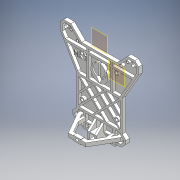
# Autodesk Inventor part: Base_v6
Saved by Autodesk Inventor 2016 (Build 200138000, 138)
## iProperties
Created: 2015-10-26
Part Number: Base_v6
Material: Generic
Document SubType Name: Modeling
Designer: Jared
Density: 1 g/cm^3
Appearance: Default
Author: Jared
Autodesk Inventor part; units mm, degrees
(part 1 of 2)
ref_plane "YZ Plane" through (0, 0, 0) normal (1, 0, 0) x (0, 1, 0)
ref_plane "XZ Plane" through (0, 0, 0) normal (0, 1, 0) x (-1, 0, 0)
ref_plane "XY Plane" through (0, 0, 0) normal (0, 0, 1) x (1, 0, 0)
sketch "Block1" plane through (0, 0, 0) normal (0, 0, 1) x (1, 0, 0)
  line L0 (52, 0) -> (42, 0)
  line L1 (52, 0) -> (56.9992, -4.9992)
  line L2 (52, 0) -> (59.07, 0) construction
  line L3 (56.9992, -4.9992) -> (56.9992, -14.9992)
  point P0 (53.472, -3.4612)
sketch "OuterRim" plane through (0, 0, 0) normal (0, 0, 1) x (1, 0, 0)
  line L0 (39.5, 1) -> (24.5001, -13.9999)
  line L1 (24.5001, -13.9999) -> (0.0001, -13.9999)
  line L2 (54.5031, -13.9999) -> (32.0031, -52.971)
  line L3 (32.0031, -52.971) -> (32.0031, -111.471)
  line L4 (32.0031, -111.471) -> (37.0024, -116.4702)
  line L5 (37.0024, -121.4734) -> (32.0002, -126.4756)
  line L6 (37.0024, -121.4734) -> (37.0024, -116.4702)
  line L7 (22.0011, -131.4748) -> (0.0003, -131.4748)
  line L8 (32.0002, -126.4756) -> (30.5003, -127.9756)
  line L9 (30.5003, -127.9756) -> (25.5003, -127.9756)
  line L10 (25.5003, -127.9756) -> (22.0011, -131.4748)
  line L11 (-36.9986, -121.4763) -> (-31.9993, -126.4756)
  line L12 (-36.9986, -121.4763) -> (-36.9986, -116.4706)
  line L13 (-31.9993, -126.4756) -> (-30.4993, -127.9756)
  line L14 (-22.0002, -131.4748) -> (0.0003, -131.4748)
  line L15 (-31.999, -111.471) -> (-36.9986, -116.4706)
  line L16 (-30.4993, -127.9756) -> (-25.4993, -127.9756)
  line L17 (-25.4993, -127.9756) -> (-22.0002, -131.4748)
  line L18 (-31.999, -52.971) -> (-31.999, -111.471)
  line L19 (-39.4997, 1) -> (-24.4999, -13.9999)
  line L20 (-24.4999, -13.9999) -> (0.0001, -13.9999)
  line L21 (-54.499, -13.9999) -> (-31.999, -52.971)
  line L22 (49.5, 1) -> (39.5, 1)
  line L23 (49.5, 1) -> (54.4992, -3.9992)
  line L24 (49.5, 1) -> (56.57, 1) construction
  line L25 (54.4992, -3.9992) -> (54.4992, -13.9992)
  line L26 (-49.4997, 1) -> (-39.4997, 1)
  line L27 (-49.4997, 1) -> (-54.499, -3.9992)
  line L28 (-49.4997, 1) -> (-56.5697, 1) construction
  line L29 (-54.499, -3.9992) -> (-54.499, -13.9992)
  point P0 (0.0001, -89.0989)
sketch "OuterRim1" plane through (0, 0, 0) normal (0, 0, 1) x (1, 0, 0)
  line L0 (-39.4997, 1) -> (-24.4999, -13.9998)
  line L1 (-24.4999, -13.9998) -> (0.0001, -13.9998)
  line L2 (-54.499, -13.9998) -> (-31.999, -52.971)
  line L3 (-31.999, -52.971) -> (-31.999, -111.471)
  line L4 (-31.999, -111.471) -> (-36.9986, -116.4706)
  line L5 (-36.9986, -121.4763) -> (-31.9993, -126.4756)
  line L6 (-36.9986, -121.4763) -> (-36.9986, -116.4706)
  line L7 (-22.0002, -131.4747) -> (0.0003, -131.4747)
  line L8 (-31.9993, -126.4756) -> (-30.4993, -127.9756)
  line L9 (-30.4993, -127.9756) -> (-25.4993, -127.9756)
  line L10 (-25.4993, -127.9756) -> (-22.0002, -131.4747)
  line L11 (39.5, 1) -> (24.5001, -13.9998)
  line L12 (24.5001, -13.9998) -> (0.0001, -13.9998)
  line L13 (32.0002, -126.4756) -> (30.5003, -127.9756)
  line L14 (30.5003, -127.9756) -> (25.5003, -127.9756)
  line L15 (25.5003, -127.9756) -> (22.0011, -131.4747)
  line L16 (54.5031, -13.9998) -> (32.0031, -52.971)
  line L17 (32.0031, -52.971) -> (32.0031, -111.471)
  line L18 (32.0031, -111.471) -> (37.0024, -116.4702)
  line L19 (37.0024, -121.4734) -> (32.0002, -126.4756)
  line L20 (37.0024, -121.4734) -> (37.0024, -116.4702)
  line L21 (22.0011, -131.4747) -> (0.0003, -131.4747)
  line L22 (49.5, 1) -> (39.5, 1)
  line L23 (49.5, 1) -> (54.5031, -3.9992)
  line L24 (54.5031, -3.9992) -> (54.5031, -13.9998)
  line L25 (-49.4997, 1) -> (-39.4997, 1)
  line L26 (-49.4997, 1) -> (-54.499, -3.9992)
  line L27 (-54.499, -3.9992) -> (-54.499, -13.9998)
  point P0 (0.0008, -71.4203)
sketch "outerrim2" plane through (0, 0, 0) normal (0, 0, 1) x (1, 0, 0)
  line L0 (49.5, 1) -> (39.5, 1)
  line L1 (49.5, 1) -> (54.5012, -3.9973)
  line L2 (54.5012, -3.9973) -> (54.5012, -13.9979)
  line L3 (-49.4997, 1) -> (-39.4997, 1)
  line L4 (-49.4997, 1) -> (-54.499, -3.9992)
  line L5 (-54.499, -3.9992) -> (-54.499, -13.9998)
  line L6 (-39.4997, 1) -> (-24.4999, -13.9998)
  line L7 (-24.4999, -13.9998) -> (0.0001, -13.9998)
  line L8 (-54.499, -13.9998) -> (-31.999, -52.971)
  line L9 (-31.999, -101.471) -> (-36.9986, -106.4706)
  line L10 (-36.9986, -111.4763) -> (-31.9993, -116.4756)
  line L11 (-36.9986, -111.4763) -> (-36.9986, -106.4706)
  line L12 (-22.0002, -121.4747) -> (0.0003, -121.4747)
  line L13 (-31.9993, -116.4756) -> (-30.4993, -117.9756)
  line L14 (-30.4993, -117.9756) -> (-25.4993, -117.9756)
  line L15 (-25.4993, -117.9756) -> (-22.0002, -121.4747)
  line L16 (39.5, 1) -> (24.5001, -13.9998)
  line L17 (24.5001, -13.9998) -> (0.0001, -13.9998)
  line L18 (32.0002, -116.4756) -> (30.5003, -117.9756)
  line L19 (30.5003, -117.9756) -> (25.5003, -117.9756)
  line L20 (25.5003, -117.9756) -> (22.0011, -121.4747)
  line L21 (54.5012, -13.9979) -> (32.0031, -52.971)
  line L22 (32.0031, -101.471) -> (37.0024, -106.4702)
  line L23 (37.0024, -111.4734) -> (32.0002, -116.4756)
  line L24 (37.0024, -111.4734) -> (37.0024, -106.4702)
  line L25 (22.0011, -121.4747) -> (0.0003, -121.4747)
  line L26 (-31.999, -52.971) -> (-31.999, -101.471)
  line L27 (32.0031, -52.971) -> (32.0031, -101.471)
  point P0 (0.0009, -67.4302)
sketch "Sketch1" plane through (0, 0, 0) normal (0, 1, 0) x (-1, 0, 0)
  line L0 (24.9992, -101.4702) -> (24.9992, -106.4702)
  line L1 (24.9992, -101.4702) -> (29.9992, -101.4702)
  line L2 (29.9992, -101.4702) -> (29.9992, -106.4702)
  line L3 (29.9992, -106.4702) -> (24.9992, -106.4702)
  line L4 (22.0008, -108.476) -> (24.9999, -111.4752)
  line L5 (22.0008, -114.4744) -> (24.9999, -111.4752)
  line L6 (33.9992, -105.2276) -> (30.7516, -108.4752)
  line L7 (33.9992, -103.2094) -> (33.9992, -105.2276)
  line L8 (29.9986, -51.0238) -> (29.1311, -53.1497)
  line L9 (51.4221, -5.197) -> (51.4221, -13.955)
  line L10 (48.1802, -1.9551) -> (51.4221, -5.197)
  line L11 (26.5443, -16.0763) -> (40.6655, -1.9551)
  line L12 (40.6655, -1.9551) -> (48.1802, -1.9551)
  line L13 (24.423, -16.955) -> (26.5443, -16.0763)
  line L14 (0.0001, -13.9999) -> (3.0001, -13.9999) construction
  line L15 (15.5025, -107.9762) -> (12.7427, -110.1594)
  line L16 (6.5073, -114.9942) -> (11.0731, -111.4803)
  line L17 (13.1989, -114.9663) -> (15.569, -114.9604)
  line L18 (13.1989, -114.9663) -> (9.927, -114.9744)
  line L19 (9.927, -114.9744) -> (12.7467, -112.7943)
  line L20 (9.927, -114.9744) -> (13.4912, -114.9744) construction
  line L21 (18.978, -107.9762) -> (14.4463, -111.4804)
  line L22 (14.4463, -111.4804) -> (18.978, -114.9745)
  line L23 (12.7427, -110.1594) -> (9.9014, -107.9762)
  line L24 (11.0731, -111.4803) -> (6.5073, -107.976)
  line L25 (12.7467, -112.7943) -> (15.569, -114.9604)
  line L26 (22.0008, -106.476) -> (23.9999, -108.4752)
  line L27 (22.0008, -108.476) -> (22.0008, -114.4744)
  line L28 (18.978, -107.9762) -> (18.978, -114.9745)
  line L29 (6.5073, -107.976) -> (6.5073, -114.9942)
  line L30 (3.5, -108.0056) -> (3.5, -115.0056)
  circle A0 centre (39.4726, -5.9876) radius 1.1
  circle A1 centre (30.4217, -15.0386) radius 1.1
  line L31 (30.7516, -108.4752) -> (29.2517, -109.9752)
  line L32 (23.9999, -108.4752) -> (25.4999, -109.9752)
  line L33 (25.4999, -109.9752) -> (29.2517, -109.9752)
  line L34 (33.9992, -103.2094) -> (29, -98.2258)
  line L35 (29, -98.2258) -> (29, -96.471)
  circle A2 centre (23.9999, -27) radius 1.5
  circle A3 centre (23.9999, -83) radius 1.5
  line L36 (9.5, -55.971) -> (18.4788, -64.9632)
  line L37 (20.0067, -66.4933) -> (29, -75.5)
  line L38 (7.9989, -57.4721) -> (16.9989, -66.4855)
  line L39 (18.5056, -67.9944) -> (27.4978, -77)
  line L40 (27.471, -55.971) -> (18.4788, -64.9632)
  line L41 (20.0067, -66.4933) -> (29, -57.5)
  line L42 (29, -57.5) -> (29, -75.5)
  line L43 (27.471, -55.971) -> (9.5, -55.971)
  line L44 (6.5, -55.971) -> (0.0001, -55.971)
  line L45 (29.1311, -53.1497) -> (18.1317, -53.2075)
  line L46 (15, -52.971) -> (0.0001, -52.971)
  line L47 (24.423, -16.955) -> (18, -16.955)
  line L48 (15, -16.9999) -> (0.0001, -16.9999)
  line L49 (22.0008, -106.476) -> (22.0008, -96.471)
  line L50 (19.0008, -106.476) -> (19.0008, -96.471)
  line L51 (3.5, -106.476) -> (3.5, -96.471)
  line L52 (6.5, -106.476) -> (6.5, -96.471)
  line L53 (6.5, -106.476) -> (19.0008, -106.476)
  line L54 (22.0008, -96.471) -> (29, -96.471)
  line L55 (19.0008, -96.471) -> (6.5, -96.471)
  line L56 (18, -28.1451) -> (18.1317, -53.2075)
  line L57 (15, -28) -> (15, -52.971)
  line L58 (43.2847, -28.1039) -> (29.9986, -51.0238)
  line L59 (-24.999, -101.4702) -> (-24.999, -106.4702)
  line L60 (-24.999, -101.4702) -> (-29.999, -101.4702)
  line L61 (-29.999, -101.4702) -> (-29.999, -106.4702)
  line L62 (-29.999, -106.4702) -> (-24.999, -106.4702)
  line L63 (-22.0005, -108.476) -> (-24.9996, -111.4752)
  line L64 (-22.0005, -114.4744) -> (-24.9996, -111.4752)
  line L65 (-33.999, -105.2276) -> (-30.7514, -108.4752)
  line L66 (-33.999, -103.2094) -> (-33.999, -105.2276)
  line L67 (-29.8784, -50.8497) -> (-28.9997, -52.971)
  line L68 (-51.4218, -5.197) -> (-51.4218, -13.955)
  line L69 (-48.1799, -1.9551) -> (-51.4218, -5.197)
  line L70 (-26.544, -16.0763) -> (-40.6652, -1.9551)
  line L71 (-40.6652, -1.9551) -> (-48.1799, -1.9551)
  line L72 (-24.4227, -16.955) -> (-26.544, -16.0763)
  line L73 (0.0001, -13.9999) -> (-2.9999, -13.9999) construction
  line L74 (-15.5021, -107.976) -> (-12.7423, -110.1593)
  line L75 (-6.5069, -114.9941) -> (-11.0727, -111.4802)
  line L76 (-13.1987, -114.9663) -> (-15.5687, -114.9604)
  line L77 (-13.1987, -114.9663) -> (-9.9267, -114.9744)
  line L78 (-9.9267, -114.9744) -> (-12.7464, -112.7943)
  line L79 (-9.9267, -114.9744) -> (-13.4909, -114.9744) construction
  line L80 (-18.9776, -107.976) -> (-14.4459, -111.4803)
  line L81 (-14.4459, -111.4803) -> (-18.9776, -114.9744)
  line L82 (-12.7423, -110.1593) -> (-9.901, -107.976)
  line L83 (-11.0727, -111.4802) -> (-6.5069, -107.9759)
  line L84 (-12.7464, -112.7943) -> (-15.5687, -114.9604)
  line L85 (-22.0005, -106.476) -> (-23.9996, -108.4752)
  line L86 (-22.0005, -108.476) -> (-22.0005, -114.4744)
  line L87 (-18.9776, -107.976) -> (-18.9776, -114.9744)
  line L88 (-6.5069, -107.9759) -> (-6.5069, -114.9941)
  line L89 (-3.4997, -108.0056) -> (-3.4997, -115.0056)
  circle A4 centre (-39.4723, -5.9876) radius 1.1
  circle A5 centre (-30.4214, -15.0386) radius 1.1
  line L90 (-30.7514, -108.4752) -> (-29.2514, -109.9752)
  line L91 (-23.9996, -108.4752) -> (-25.4997, -109.9752)
  line L92 (-25.4997, -109.9752) -> (-29.2514, -109.9752)
  line L93 (-33.999, -103.2094) -> (-28.9997, -98.2258)
  line L94 (-28.9997, -98.2258) -> (-28.9997, -96.471)
  circle A6 centre (-23.9996, -27) radius 1.5
  circle A7 centre (-23.9996, -83) radius 1.5
  line L95 (-9.4997, -55.971) -> (-18.4785, -64.9632)
  line L96 (-20.0064, -66.4933) -> (-28.9997, -75.5)
  line L97 (-7.9986, -57.4721) -> (-16.9986, -66.4855)
  line L98 (-18.5053, -67.9945) -> (-27.4975, -77.0001)
  line L99 (-27.4707, -55.971) -> (-18.4785, -64.9632)
  line L100 (-20.0064, -66.4933) -> (-28.9997, -57.5)
  line L101 (-28.9997, -57.5) -> (-28.9997, -75.5)
  line L102 (-27.4707, -55.971) -> (-9.4997, -55.971)
  line L103 (-6.4997, -55.971) -> (0.0001, -55.971)
  line L104 (-28.9997, -52.971) -> (-17.9997, -52.971)
  line L105 (-14.9997, -52.971) -> (0.0001, -52.971)
  line L106 (-24.4227, -16.955) -> (-17.9997, -16.955)
  line L107 (-14.9997, -16.9999) -> (0.0001, -16.9999)
  line L108 (-22.0005, -106.476) -> (-22.0005, -96.471)
  line L109 (-19.0005, -106.476) -> (-19.0005, -96.471)
  line L110 (-3.4997, -106.476) -> (-3.4997, -96.471)
  line L111 (-6.4997, -106.476) -> (-6.4997, -96.471)
  line L112 (-6.4997, -106.476) -> (-19.0005, -106.476)
  line L113 (-22.0005, -96.471) -> (-28.9997, -96.471)
  line L114 (-19.0005, -96.471) -> (-6.4997, -96.471)
  line L115 (-17.9997, -28) -> (-17.9997, -52.971)
  line L116 (-14.9997, -28) -> (-14.9997, -52.971)
  line L117 (-51.4218, -13.955) -> (-45.0449, -25)
  line L118 (-43.2848, -28) -> (-29.8784, -50.8497)
  line L119 (54.5012, -13.9979) -> (54.4973, -13.9973)
  line L120 (3.5, -115.0056) -> (-3.4997, -115.0056)
  line L121 (3.5, -96.471) -> (-3.4997, -96.471)
  line L122 (49.5, 1) -> (56.57, 1) construction
  line L123 (-49.4997, 1) -> (-56.5697, 1) construction
  line L124 (-15.5021, -107.976) -> (-9.901, -107.976)
  line L125 (15.5025, -107.9762) -> (9.9014, -107.9762)
  line L126 (-17.9997, -21) -> (-47.3543, -21)
  line L127 (-17.9997, -16.955) -> (-17.9997, -21)
  line L128 (-14.9997, -16.9999) -> (-14.9997, -21)
  line L129 (15, -21) -> (-14.9997, -21)
  line L130 (15, -16.9999) -> (15, -21)
  line L131 (18, -21) -> (18, -16.955)
  line L132 (18, -21) -> (47.3546, -21)
  line L133 (51.4221, -13.955) -> (47.3546, -21)
  line L134 (45.6012, -24.0917) -> (43.2847, -28.1039)
  line L135 (18, -28.1451) -> (18, -24.0917)
  line L136 (-17.9997, -24) -> (-45.6223, -24)
  line L137 (15, -24) -> (15, -28)
  line L138 (-14.9997, -24) -> (-14.9997, -28)
  line L139 (-17.9997, -28) -> (-17.9997, -24)
  circle A8 centre (-46.9997, -6.5) radius 2
  circle A9 centre (47, -6.5) radius 2
  circle A10 centre (-23.9996, -27) radius 3
  arc A11 (-21.0442, -83.5154) -> (-23.4842, -85.9554) centre (-23.9996, -83) ccw
  arc A12 (23.2638, -24.0917) -> (24.7361, -24.0917) centre (23.9999, -27) ccw
  arc A13 (23.4849, -85.9555) -> (21.0445, -83.515) centre (23.9999, -83) ccw
  circle A14 centre (30.4217, -15.0386) radius 2
  circle A15 centre (39.4726, -5.9876) radius 2
  circle A16 centre (-30.4214, -15.0386) radius 2
  circle A17 centre (-39.4723, -5.9876) radius 2
  line L140 (1, -29) -> (1, -42.9373)
  line L141 (-1, -29) -> (-1, -42.9372)
  line L142 (0, -50.9997) -> (-3.9281, -44.1961)
  line L143 (0, -50.9997) -> (3.9287, -44.1961)
  line L144 (-45.0449, -25) -> (-43.2848, -28)
  line L145 (-14.9997, -24) -> (15, -24)
  line L146 (-3.4997, -106.476) -> (3.5, -106.476)
  line L147 (-3.4997, -108.0056) -> (3.5, -108.0056)
  arc A18 (-9.367, -31.4996) -> (9.3679, -31.5004) centre (0.0001, -39) ccw
  arc A19 (-9.367, -31.4996) -> (-3.9281, -44.1961) centre (0.0003, -35) ccw
  arc A20 (3.9287, -44.1961) -> (9.3679, -31.5004) centre (0.0003, -35) ccw
  line L148 (-1, -29) -> (-1, -27.0628)
  line L149 (1, -29) -> (1, -27.0627)
  arc A21 (1, -42.9373) -> (1, -27.0627) centre (0.0003, -35) ccw
  arc A22 (-1, -27.0628) -> (-1, -42.9372) centre (0.0003, -35) ccw
  line L150 (49.5, 1) -> (39.5, 1)
  line L151 (49.5, 1) -> (54.5012, -3.9973)
  line L152 (54.5012, -3.9973) -> (54.5012, -13.9979)
  line L153 (-49.4997, 1) -> (-39.4997, 1)
  line L154 (-39.4997, 1) -> (-24.4999, -13.9998)
  line L155 (-24.4999, -13.9998) -> (0.0001, -13.9998)
  line L156 (-31.999, -96.471) -> (-36.9986, -101.4706)
  line L157 (-36.9986, -106.4763) -> (-31.9993, -111.4756)
  line L158 (-36.9986, -106.4763) -> (-36.9986, -101.4706)
  line L159 (-22.0002, -116.4747) -> (0.0003, -116.4747)
  line L160 (-31.9993, -111.4756) -> (-30.4993, -112.9756)
  line L161 (-30.4993, -112.9756) -> (-25.4993, -112.9756)
  line L162 (-25.4993, -112.9756) -> (-22.0002, -116.4747)
  line L163 (39.5, 1) -> (24.5001, -13.9998)
  line L164 (24.5001, -13.9998) -> (0.0001, -13.9998)
  line L165 (32.0002, -111.4756) -> (30.5003, -112.9756)
  line L166 (30.5003, -112.9756) -> (25.5003, -112.9756)
  line L167 (25.5003, -112.9756) -> (22.0011, -116.4747)
  line L168 (54.5012, -13.9979) -> (32.0031, -52.971)
  line L169 (32.0031, -96.471) -> (37.0024, -101.4702)
  line L170 (37.0024, -106.4734) -> (32.0002, -111.4756)
  line L171 (37.0024, -106.4734) -> (37.0024, -101.4702)
  line L172 (22.0011, -116.4747) -> (0.0003, -116.4747)
  line L173 (-49.4997, 1) -> (-54.499, -3.9992)
  line L174 (-54.499, -3.9992) -> (-54.499, -13.9998)
  line L175 (-54.499, -13.9998) -> (-31.999, -52.971)
  line L176 (-31.999, -52.971) -> (-31.999, -96.471)
  line L177 (32.0031, -52.971) -> (32.0031, -96.471)
  line L178 (29, -78.5022) -> (29, -91.4705)
  line L179 (-28.9997, -78.5045) -> (-28.9997, -91.4709)
  line L180 (-27.4975, -77.0001) -> (-28.9997, -78.5045)
  line L181 (-28.0288, -93.5) -> (28.0295, -93.5)
  line L182 (27.4978, -77) -> (29, -78.5022)
  line L183 (23.4849, -85.9555) -> (29, -91.4705)
  line L184 (-23.4842, -85.9554) -> (-28.9997, -91.4709)
  line L185 (-10.5143, -75.9855) -> (-28.0288, -93.5)
  line L186 (-16.9986, -66.4855) -> (-10.4934, -72.9645)
  line L187 (-8.9904, -74.4615) -> (-6.4417, -77)
  line L188 (-12.0144, -74.4855) -> (-21.0442, -83.5154)
  line L189 (-9.4997, -77.0001) -> (-10.5143, -75.9855)
  line L190 (-12.0144, -74.4855) -> (-18.5053, -67.9945)
  line L191 (-7.9986, -57.4721) -> (-1.4998, -63.9709)
  line L192 (6.5, -55.971) -> (0.0002, -62.4709)
  line L193 (-1.4998, -63.9709) -> (-10.4934, -72.9645)
  line L194 (-6.4997, -55.971) -> (0.0002, -62.4709)
  line L195 (7.9989, -57.4721) -> (1.5002, -63.9709)
  line L196 (0.0002, -65.4709) -> (-8.9904, -74.4615)
  line L197 (16.9989, -66.4855) -> (10.4938, -72.9644)
  line L198 (8.9908, -74.4614) -> (6.442, -77)
  line L199 (9.5, -77) -> (10.5147, -75.9853)
  line L200 (12.0147, -74.4853) -> (18.5056, -67.9944)
  line L201 (0.0002, -65.4709) -> (8.9908, -74.4614)
  line L202 (10.5147, -75.9853) -> (28.0295, -93.5)
  line L203 (1.5002, -63.9709) -> (10.4938, -72.9644)
  line L204 (12.0147, -74.4853) -> (21.0445, -83.515)
  line L205 (-6.4417, -77) -> (0.0002, -83.4419)
  line L206 (1.5292, -84.9709) -> (10.0584, -93.5)
  line L207 (-9.4997, -77.0001) -> (-1.5289, -84.9709)
  line L208 (0.0002, -86.4999) -> (7.0003, -93.5)
  line L209 (6.442, -77) -> (0.0002, -83.4419)
  line L210 (-1.5289, -84.9709) -> (-10.0579, -93.5)
  line L211 (9.5, -77) -> (1.5292, -84.9709)
  line L212 (0.0002, -86.4999) -> (-6.9999, -93.5)
  line L213 (18, -24.0917) -> (23.2638, -24.0917)
  line L214 (24.7361, -24.0917) -> (45.6012, -24.0917)
  constraints: 433 end point, 30 parallel, 23 centre point, 16 point on circle, 15 horizontal, 14 point on line, 13 perpendicular, 9 coincident, 8 vertical, 1 collinear, 1 equal length
ref_plane "Work Plane3" through (0, 0, 0) normal (0, -1, 0) x (1, 0, 0)
sketch "Sketch8" plane through (0, 0, 0) normal (0, -1, 0) x (1, 0, 0)
  line L0 (49.5, 1) -> (39.5, 1)
  line L1 (49.5, 1) -> (54.5012, -3.9973)
  line L2 (54.5012, -3.9973) -> (54.5012, -13.9979)
  line L3 (-49.4997, 1) -> (-39.4997, 1)
  line L4 (-49.4997, 1) -> (-54.499, -3.9992)
  line L5 (-54.499, -3.9992) -> (-54.499, -13.9999)
  line L6 (-39.4997, 1) -> (-24.4999, -13.9999)
  line L7 (-24.4999, -13.9999) -> (0.0001, -13.9999)
  line L8 (-54.499, -13.9999) -> (-31.999, -52.971)
  line L9 (-31.999, -96.471) -> (-36.9986, -101.4706)
  line L10 (-36.9986, -106.4763) -> (-31.9993, -111.4756)
  line L11 (-36.9986, -106.4763) -> (-36.9986, -101.4706)
  line L12 (-22.0002, -116.4748) -> (0.0003, -116.4748)
  line L13 (-31.9993, -111.4756) -> (-30.4993, -112.9756)
  line L14 (-30.4993, -112.9756) -> (-25.4993, -112.9756)
  line L15 (-25.4993, -112.9756) -> (-22.0002, -116.4748)
  line L16 (39.5, 1) -> (24.5001, -13.9999)
  line L17 (24.5001, -13.9999) -> (0.0001, -13.9999)
  line L18 (32.0002, -111.4756) -> (30.5003, -112.9756)
  line L19 (30.5003, -112.9756) -> (25.5003, -112.9756)
  line L20 (25.5003, -112.9756) -> (22.0011, -116.4748)
  line L21 (54.5012, -13.9979) -> (32.0031, -52.971)
  line L22 (32.0031, -96.471) -> (37.0024, -101.4702)
  line L23 (37.0024, -106.4734) -> (32.0002, -111.4756)
  line L24 (37.0024, -106.4734) -> (37.0024, -101.4702)
  line L25 (22.0011, -116.4748) -> (0.0003, -116.4748)
  line L26 (32.0031, -52.971) -> (32.0031, -96.471)
  line L27 (-31.999, -96.471) -> (-31.999, -52.971)
  point P0 (0, 0)
  constraints: 56 end point, 4 horizontal, 2 vertical, 1 parallel, 1 perpendicular
ref_plane "Work Plane8" through (23.9996, 0, -27) normal (0, -1, 0) x (1, 0, 0)
sketch "Sketch10" plane through (23.9996, 0, -27) normal (0, -1, 0) x (1, 0, 0)
  circle A0 centre (0.0003, 0) radius 1.5 projected
  circle A1 centre (0.0003, 0) radius 1.5
  circle A2 centre (-47.9993, 0) radius 1.5 projected
  circle A3 centre (-47.9993, 0) radius 1.5
  circle A4 centre (-47.9993, 0) radius 2.9998
  circle A5 centre (-47.9996, -56) radius 3 projected
  circle A6 centre (-47.9996, -56) radius 1.5001
  circle A7 centre (-47.9996, -56) radius 3
  arc A8 (-0.0236, -53.0001) -> (0.0236, -53.0001) centre (0, -56) ccw projected
  circle A9 centre (0, -56) radius 1.5
  circle A10 centre (0, -56) radius 3
  circle A11 centre (0.0003, 0) radius 3
  circle A12 centre (0.0003, 0) radius 1.5
  point P0 (-23.9996, 27)
  dimension "d136" = 3
  constraints: 9 centre point, 9 coincident
  measures "d136" diameter of A1
sketch "Sketch20" plane through (0, 0, 0) normal (0, -1, 0) x (1, 0, 0)
  line L0 (24.9992, -101.4702) -> (24.9992, -106.4702)
  line L1 (24.9992, -101.4702) -> (29.9992, -101.4702)
  line L2 (29.9992, -101.4702) -> (29.9992, -106.4702)
  line L3 (29.9992, -106.4702) -> (24.9992, -106.4702)
  line L4 (22.0008, -108.476) -> (24.9999, -111.4752)
  line L5 (22.0008, -114.4744) -> (24.9999, -111.4752)
  line L6 (33.9992, -105.2276) -> (30.7516, -108.4752)
  line L7 (33.9992, -103.2094) -> (33.9992, -105.2276)
  line L8 (29.9986, -51.0238) -> (29.1311, -53.1497)
  line L9 (51.4221, -5.197) -> (51.4221, -13.955)
  line L10 (48.1802, -1.9551) -> (51.4221, -5.197)
  line L11 (26.5443, -16.0763) -> (40.6655, -1.9551)
  line L12 (40.6655, -1.9551) -> (48.1802, -1.9551)
  line L13 (24.423, -16.955) -> (26.5443, -16.0763)
  line L14 (0.0001, -13.9999) -> (3.0001, -13.9999) construction
  line L15 (15.5025, -107.9762) -> (12.7427, -110.1594)
  line L16 (6.5073, -114.9942) -> (11.0731, -111.4803)
  line L17 (13.1989, -114.9663) -> (15.569, -114.9604)
  line L18 (13.1989, -114.9663) -> (9.927, -114.9744)
  line L19 (9.927, -114.9744) -> (12.7467, -112.7943)
  line L20 (9.927, -114.9744) -> (13.4912, -114.9744) construction
  line L21 (18.978, -107.9762) -> (14.4463, -111.4804)
  line L22 (14.4463, -111.4804) -> (18.978, -114.9745)
  line L23 (12.7427, -110.1594) -> (9.9014, -107.9762)
  line L24 (11.0731, -111.4803) -> (6.5073, -107.976)
  line L25 (12.7467, -112.7943) -> (15.569, -114.9604)
  line L26 (22.0008, -106.476) -> (23.9999, -108.4752)
  line L27 (22.0008, -108.476) -> (22.0008, -114.4744)
  line L28 (18.978, -107.9762) -> (18.978, -114.9745)
  line L29 (6.5073, -107.976) -> (6.5073, -114.9942)
  line L30 (3.5, -108.0056) -> (3.5, -115.0056)
  circle A0 centre (39.4726, -5.9876) radius 1.1
  circle A1 centre (30.4217, -15.0386) radius 1.1
  line L31 (30.7516, -108.4752) -> (29.2517, -109.9752)
  line L32 (23.9999, -108.4752) -> (25.4999, -109.9752)
  line L33 (25.4999, -109.9752) -> (29.2517, -109.9752)
  line L34 (33.9992, -103.2094) -> (29, -98.2258)
  line L35 (29, -98.2258) -> (29, -96.471)
  circle A2 centre (23.9999, -27) radius 1.5
  circle A3 centre (23.9999, -83) radius 1.5
  line L36 (9.5, -55.971) -> (18.4788, -64.9632)
  line L37 (20.0067, -66.4933) -> (29, -75.5)
  line L38 (7.9989, -57.4721) -> (16.9989, -66.4855)
  line L39 (18.5056, -67.9944) -> (27.4978, -77)
  line L40 (27.471, -55.971) -> (18.4788, -64.9632)
  line L41 (20.0067, -66.4933) -> (29, -57.5)
  line L42 (29, -57.5) -> (29, -75.5)
  line L43 (27.471, -55.971) -> (9.5, -55.971)
  line L44 (6.5, -55.971) -> (0.0001, -55.971)
  line L45 (29.1311, -53.1497) -> (18.1317, -53.2075)
  line L46 (15, -52.971) -> (0.0001, -52.971)
  line L47 (24.423, -16.955) -> (18, -16.955)
  line L48 (15, -16.9999) -> (0.0001, -16.9999)
  line L49 (22.0008, -106.476) -> (22.0008, -96.471)
  line L50 (19.0008, -106.476) -> (19.0008, -96.471)
  line L51 (3.5, -106.476) -> (3.5, -96.471)
  line L52 (6.5, -106.476) -> (6.5, -96.471)
  line L53 (6.5, -106.476) -> (19.0008, -106.476)
  line L54 (22.0008, -96.471) -> (29, -96.471)
  line L55 (19.0008, -96.471) -> (6.5, -96.471)
  line L56 (18, -28.1451) -> (18.1317, -53.2075)
  line L57 (15, -28) -> (15, -52.971)
  line L58 (43.2847, -28.1039) -> (29.9986, -51.0238)
  line L59 (-15.5021, -107.976) -> (-12.7423, -110.1593)
  line L60 (-12.7423, -110.1593) -> (-9.901, -107.976)
  line L61 (-33.999, -103.2094) -> (-33.999, -105.2276)
  line L62 (-33.999, -105.2276) -> (-30.7514, -108.4752)
  line L63 (-24.999, -101.4702) -> (-24.999, -106.4702)
  line L64 (-6.4997, -106.476) -> (-19.0005, -106.476)
  line L65 (-19.0005, -106.476) -> (-19.0005, -96.471)
  line L66 (-6.4997, -106.476) -> (-6.4997, -96.471)
  line L67 (-3.4997, -106.476) -> (-3.4997, -96.471)
  line L68 (-19.0005, -96.471) -> (-6.4997, -96.471)
  line L69 (-6.5069, -114.9941) -> (-11.0727, -111.4802)
  line L70 (-13.1987, -114.9663) -> (-15.5687, -114.9604)
  line L71 (-13.1987, -114.9663) -> (-9.9267, -114.9744)
  line L72 (-18.9776, -107.976) -> (-14.4459, -111.4803)
  line L73 (-14.4459, -111.4803) -> (-18.9776, -114.9744)
  line L74 (-18.9776, -107.976) -> (-18.9776, -114.9744)
  line L75 (-3.4997, -108.0056) -> (-3.4997, -115.0056)
  line L76 (-12.7464, -112.7943) -> (-15.5687, -114.9604)
  line L77 (-9.9267, -114.9744) -> (-13.4909, -114.9744) construction
  line L78 (-9.9267, -114.9744) -> (-12.7464, -112.7943)
  line L79 (-6.5069, -107.9759) -> (-6.5069, -114.9941)
  line L80 (-11.0727, -111.4802) -> (-6.5069, -107.9759)
  line L81 (-24.999, -101.4702) -> (-29.999, -101.4702)
  line L82 (-29.999, -101.4702) -> (-29.999, -106.4702)
  line L83 (-29.999, -106.4702) -> (-24.999, -106.4702)
  line L84 (-30.7514, -108.4752) -> (-29.2514, -109.9752)
  line L85 (-33.999, -103.2094) -> (-28.9997, -98.2258)
  line L86 (-25.4997, -109.9752) -> (-29.2514, -109.9752)
  line L87 (-22.0005, -114.4744) -> (-24.9996, -111.4752)
  line L88 (-22.0005, -108.476) -> (-22.0005, -114.4744)
  line L89 (-23.9996, -108.4752) -> (-25.4997, -109.9752)
  line L90 (-22.0005, -108.476) -> (-24.9996, -111.4752)
  line L91 (-22.0005, -106.476) -> (-23.9996, -108.4752)
  line L92 (-22.0005, -106.476) -> (-22.0005, -96.471)
  line L93 (-22.0005, -96.471) -> (-28.9997, -96.471)
  line L94 (-28.9997, -98.2258) -> (-28.9997, -96.471)
  circle A4 centre (-23.9996, -83) radius 1.5
  line L95 (-18.5053, -67.9945) -> (-27.4975, -77.0001)
  line L96 (-20.0064, -66.4933) -> (-28.9997, -75.5)
  line L97 (-28.9997, -57.5) -> (-28.9997, -75.5)
  line L98 (-20.0064, -66.4933) -> (-28.9997, -57.5)
  line L99 (-27.4707, -55.971) -> (-18.4785, -64.9632)
  line L100 (-27.4707, -55.971) -> (-9.4997, -55.971)
  line L101 (-9.4997, -55.971) -> (-18.4785, -64.9632)
  line L102 (-7.9986, -57.4721) -> (-16.9986, -66.4855)
  line L103 (-6.4997, -55.971) -> (0.0001, -55.971)
  line L104 (-51.4218, -5.197) -> (-51.4218, -13.955)
  line L105 (-48.1799, -1.9551) -> (-51.4218, -5.197)
  line L106 (-26.544, -16.0763) -> (-40.6652, -1.9551)
  line L107 (-40.6652, -1.9551) -> (-48.1799, -1.9551)
  line L108 (-24.4227, -16.955) -> (-26.544, -16.0763)
  circle A5 centre (-39.4723, -5.9876) radius 1.1
  circle A6 centre (-30.4214, -15.0386) radius 1.1
  line L109 (-24.4227, -16.955) -> (-17.9997, -16.955)
  line L110 (-51.4218, -13.955) -> (-45.0449, -25)
  line L111 (-29.8784, -50.8497) -> (-28.9997, -52.971)
  line L112 (0.0001, -13.9999) -> (-2.9999, -13.9999) construction
  circle A7 centre (-23.9996, -27) radius 1.5
  line L113 (-28.9997, -52.971) -> (-17.9997, -52.971)
  line L114 (-14.9997, -52.971) -> (0.0001, -52.971)
  line L115 (-14.9997, -28) -> (-14.9997, -52.971)
  line L116 (-17.9997, -28) -> (-17.9997, -52.971)
  line L117 (-43.2848, -28) -> (-29.8784, -50.8497)
  line L118 (-14.9997, -16.9999) -> (0.0001, -16.9999)
  line L119 (54.5012, -13.9979) -> (54.4973, -13.9973)
  line L120 (3.5, -115.0056) -> (-3.4997, -115.0056)
  line L121 (3.5, -96.471) -> (-3.4997, -96.471)
  line L122 (49.5, 1) -> (56.57, 1) construction
  line L123 (-49.4997, 1) -> (-56.5697, 1) construction
  line L124 (-15.5021, -107.976) -> (-9.901, -107.976)
  line L125 (15.5025, -107.9762) -> (9.9014, -107.9762)
  line L126 (-17.9997, -21) -> (-47.3543, -21)
  line L127 (-17.9997, -16.955) -> (-17.9997, -21)
  line L128 (-14.9997, -16.9999) -> (-14.9997, -21)
  line L129 (15, -21) -> (-14.9997, -21)
  line L130 (15, -16.9999) -> (15, -21)
  line L131 (18, -21) -> (18, -16.955)
  line L132 (18, -21) -> (47.3546, -21)
  line L133 (51.4221, -13.955) -> (47.3546, -21)
  line L134 (45.6012, -24.0917) -> (43.2847, -28.1039)
  line L135 (18, -28.1451) -> (18, -24.0917)
  line L136 (-17.9997, -24) -> (-45.6223, -24)
  line L137 (15, -24) -> (15, -28)
  line L138 (-14.9997, -24) -> (-14.9997, -28)
  line L139 (-17.9997, -28) -> (-17.9997, -24)
  circle A8 centre (-46.9997, -6.5) radius 2
  circle A9 centre (47, -6.5) radius 2
  circle A10 centre (-23.9996, -27) radius 3
  arc A11 (-21.0442, -83.5154) -> (-23.4842, -85.9554) centre (-23.9996, -83) ccw
  arc A12 (23.2638, -24.0917) -> (24.7361, -24.0917) centre (23.9999, -27) ccw
  arc A13 (23.4849, -85.9555) -> (21.0445, -83.515) centre (23.9999, -83) ccw
  circle A14 centre (30.4217, -15.0386) radius 2
  circle A15 centre (39.4726, -5.9876) radius 2
  circle A16 centre (-30.4214, -15.0386) radius 2
  circle A17 centre (-39.4723, -5.9876) radius 2
  line L140 (1, -29) -> (1, -42.9373)
  line L141 (-1, -29) -> (-1, -42.9372)
  line L142 (0, -50.9997) -> (-3.9281, -44.1961)
  line L143 (0, -50.9997) -> (3.9287, -44.1961)
  line L144 (-45.0449, -25) -> (-43.2848, -28)
  line L145 (-14.9997, -24) -> (15, -24)
  line L146 (-3.4997, -106.476) -> (3.5, -106.476)
  line L147 (-3.4997, -108.0056) -> (3.5, -108.0056)
  arc A18 (-9.367, -31.4996) -> (9.3679, -31.5004) centre (0.0001, -39) ccw
  arc A19 (-9.367, -31.4996) -> (-3.9281, -44.1961) centre (0.0003, -35) ccw
  arc A20 (3.9287, -44.1961) -> (9.3679, -31.5004) centre (0.0003, -35) ccw
  line L148 (-1, -29) -> (-1, -27.0628)
  line L149 (1, -29) -> (1, -27.0627)
  arc A21 (1, -42.9373) -> (1, -27.0627) centre (0.0003, -35) ccw
  arc A22 (-1, -27.0628) -> (-1, -42.9372) centre (0.0003, -35) ccw
  line L150 (49.5, 1) -> (39.5, 1)
  line L151 (49.5, 1) -> (54.5012, -3.9973)
  line L152 (54.5012, -3.9973) -> (54.5012, -13.9979)
  line L153 (-49.4997, 1) -> (-39.4997, 1)
  line L154 (-39.4997, 1) -> (-24.4999, -13.9998)
  line L155 (-24.4999, -13.9998) -> (0.0001, -13.9998)
  line L156 (-31.999, -96.471) -> (-36.9986, -101.4706)
  line L157 (-36.9986, -106.4763) -> (-31.9993, -111.4756)
  line L158 (-36.9986, -106.4763) -> (-36.9986, -101.4706)
  line L159 (-22.0002, -116.4747) -> (0.0003, -116.4747)
  line L160 (-31.9993, -111.4756) -> (-30.4993, -112.9756)
  line L161 (-30.4993, -112.9756) -> (-25.4993, -112.9756)
  line L162 (-25.4993, -112.9756) -> (-22.0002, -116.4747)
  line L163 (39.5, 1) -> (24.5001, -13.9998)
  line L164 (24.5001, -13.9998) -> (0.0001, -13.9998)
  line L165 (32.0002, -111.4756) -> (30.5003, -112.9756)
  line L166 (30.5003, -112.9756) -> (25.5003, -112.9756)
  line L167 (25.5003, -112.9756) -> (22.0011, -116.4747)
  line L168 (54.5012, -13.9979) -> (32.0031, -52.971)
  line L169 (32.0031, -96.471) -> (37.0024, -101.4702)
  line L170 (37.0024, -106.4734) -> (32.0002, -111.4756)
  line L171 (37.0024, -106.4734) -> (37.0024, -101.4702)
  line L172 (22.0011, -116.4747) -> (0.0003, -116.4747)
  line L173 (-49.4997, 1) -> (-54.499, -3.9992)
  line L174 (-54.499, -3.9992) -> (-54.499, -13.9998)
  line L175 (-54.499, -13.9998) -> (-31.999, -52.971)
  line L176 (-31.999, -52.971) -> (-31.999, -96.471)
  line L177 (32.0031, -52.971) -> (32.0031, -96.471)
  line L178 (29, -78.5022) -> (29, -91.4705)
  line L179 (-28.9997, -78.5045) -> (-28.9997, -91.4709)
  line L180 (-27.4975, -77.0001) -> (-28.9997, -78.5045)
  line L181 (-28.0288, -93.5) -> (28.0295, -93.5)
  line L182 (27.4978, -77) -> (29, -78.5022)
  line L183 (23.4849, -85.9555) -> (29, -91.4705)
  line L184 (-23.4842, -85.9554) -> (-28.9997, -91.4709)
  line L185 (-10.5143, -75.9855) -> (-28.0288, -93.5)
  line L186 (-16.9986, -66.4855) -> (-10.4934, -72.9645)
  line L187 (-8.9904, -74.4615) -> (-6.4417, -77)
  line L188 (-12.0144, -74.4855) -> (-21.0442, -83.5154)
  line L189 (-9.4997, -77.0001) -> (-10.5143, -75.9855)
  line L190 (-12.0144, -74.4855) -> (-18.5053, -67.9945)
  line L191 (-7.9986, -57.4721) -> (-1.4998, -63.9709)
  line L192 (6.5, -55.971) -> (0.0002, -62.4709)
  line L193 (-1.4998, -63.9709) -> (-10.4934, -72.9645)
  line L194 (-6.4997, -55.971) -> (0.0002, -62.4709)
  line L195 (7.9989, -57.4721) -> (1.5002, -63.9709)
  line L196 (0.0002, -65.4709) -> (-8.9904, -74.4615)
  line L197 (16.9989, -66.4855) -> (10.4938, -72.9644)
  line L198 (8.9908, -74.4614) -> (6.442, -77)
  line L199 (9.5, -77) -> (10.5147, -75.9853)
  line L200 (12.0147, -74.4853) -> (18.5056, -67.9944)
  line L201 (0.0002, -65.4709) -> (8.9908, -74.4614)
  line L202 (10.5147, -75.9853) -> (28.0295, -93.5)
  line L203 (1.5002, -63.9709) -> (10.4938, -72.9644)
  line L204 (12.0147, -74.4853) -> (21.0445, -83.515)
  line L205 (-6.4417, -77) -> (0.0002, -83.4419)
  line L206 (1.5292, -84.9709) -> (10.0584, -93.5)
  line L207 (-9.4997, -77.0001) -> (-1.5289, -84.9709)
  line L208 (0.0002, -86.4999) -> (7.0003, -93.5)
  line L209 (6.442, -77) -> (0.0002, -83.4419)
  line L210 (-1.5289, -84.9709) -> (-10.0579, -93.5)
  line L211 (9.5, -77) -> (1.5292, -84.9709)
  line L212 (0.0002, -86.4999) -> (-6.9999, -93.5)
  line L213 (18, -24.0917) -> (23.2638, -24.0917)
  line L214 (24.7361, -24.0917) -> (45.6012, -24.0917)
  point P0 (0, 0)
  constraints: 433 end point, 30 parallel, 23 centre point, 16 point on circle, 15 horizontal, 14 point on line, 13 perpendicular, 9 coincident, 8 vertical, 1 collinear, 1 equal length
extrude "Extrusion22" add sketch "Sketch8" against normal blind 5
extrude "Extrusion23" cut sketch "Sketch1" along normal blind 4 contours L4 L5 L27 | L6 L31 L33 L32 L26 L49 L54 L35 L34 L7 | L8 L45 L56 L135 L213 A12 L214 L134 L58 | L9 L133 L132 L131 L47 L13 L11 L12 L10 | L15 L23 L125 | L29 L24 L16 | L18 L19 L25 L17 | L28 L22 L21 | L43 L40 L36 | L41 L42 L37 | L38 L197 L203 L195 | L39 L182 L178 L183 A13 L204 L200 | L192 L194 L103 L44 | L46 L105 L116 L138 L145 L137 L57 | L130 L129 L128 L107 L48 | L53 L52 L55 L50 | L86 L64 L63 | L66 L93 L94 L113 L108 L85 L91 L92 L90 L65 | L118 L144 L117 L136 L139 L115 L104 L67 | L69 L71 L70 L72 L106 L127 L126 L117 L68 | L124 L82 L74 | L75 L83 L88 | L76 L84 L78 L77 | L80 L81 L87 | L95 L99 L102 | L96 L101 L100 | L191 L193 L186 L97 | L190 L188 A11 L184 L179 L180 L98 | L109 L114 L111 L112 | L185 L189 L207 L210 L181 | L212 L208 L181 | L206 L211 L199 L202 L181 | L196 L201 L198 L209 L205 L187
extrude "Extrusion24" cut sketch "Sketch10" against normal blind 5 contours A0 | A2 | A6 | A9
extrude "Extrusion25" cut sketch "Sketch20" against normal blind 5 contours L30 L120 L75 L147 | L146 L67 L121 L51
sketch "Sketch22" plane through (0, 0, 0) normal (0, -1, 0) x (1, 0, 0)
  line L0 (24.9992, -101.4702) -> (24.9992, -106.4702)
  line L1 (24.9992, -101.4702) -> (29.9992, -101.4702)
  line L2 (29.9992, -101.4702) -> (29.9992, -106.4702)
  line L3 (29.9992, -106.4702) -> (24.9992, -106.4702)
  line L4 (22.0008, -108.476) -> (24.9999, -111.4752)
  line L5 (22.0008, -114.4744) -> (24.9999, -111.4752)
  line L6 (33.9992, -105.2276) -> (30.7516, -108.4752)
  line L7 (33.9992, -103.2094) -> (33.9992, -105.2276)
  line L8 (29.9986, -51.0238) -> (29.1311, -53.1497)
  line L9 (51.4221, -5.197) -> (51.4221, -13.955)
  line L10 (48.1802, -1.9551) -> (51.4221, -5.197)
  line L11 (26.5443, -16.0763) -> (40.6655, -1.9551)
  line L12 (40.6655, -1.9551) -> (48.1802, -1.9551)
  line L13 (24.423, -16.955) -> (26.5443, -16.0763)
  line L14 (0.0001, -13.9999) -> (3.0001, -13.9999) construction
  line L15 (15.5025, -107.9762) -> (12.7427, -110.1594)
  line L16 (6.5073, -114.9942) -> (11.0731, -111.4803)
  line L17 (13.1989, -114.9663) -> (15.569, -114.9604)
  line L18 (13.1989, -114.9663) -> (9.927, -114.9744)
  line L19 (9.927, -114.9744) -> (12.7467, -112.7943)
  line L20 (9.927, -114.9744) -> (13.4912, -114.9744) construction
  line L21 (18.978, -107.9762) -> (14.4463, -111.4804)
  line L22 (14.4463, -111.4804) -> (18.978, -114.9745)
  line L23 (12.7427, -110.1594) -> (9.9014, -107.9762)
  line L24 (11.0731, -111.4803) -> (6.5073, -107.976)
  line L25 (12.7467, -112.7943) -> (15.569, -114.9604)
  line L26 (22.0008, -106.476) -> (23.9999, -108.4752)
  line L27 (22.0008, -108.476) -> (22.0008, -114.4744)
  line L28 (18.978, -107.9762) -> (18.978, -114.9745)
  line L29 (6.5073, -107.976) -> (6.5073, -114.9942)
  line L30 (3.5, -108.0056) -> (3.5, -115.0056)
  circle A0 centre (39.4726, -5.9876) radius 1.1
  circle A1 centre (30.4217, -15.0386) radius 1.1
  line L31 (30.7516, -108.4752) -> (29.2517, -109.9752)
  line L32 (23.9999, -108.4752) -> (25.4999, -109.9752)
  line L33 (25.4999, -109.9752) -> (29.2517, -109.9752)
  line L34 (33.9992, -103.2094) -> (29, -98.2258)
  line L35 (29, -98.2258) -> (29, -96.471)
  circle A2 centre (23.9999, -27) radius 1.5
  circle A3 centre (23.9999, -83) radius 1.5
  line L36 (9.5, -55.971) -> (18.4788, -64.9632)
  line L37 (20.0067, -66.4933) -> (29, -75.5)
  line L38 (7.9989, -57.4721) -> (16.9989, -66.4855)
  line L39 (18.5056, -67.9944) -> (27.4978, -77)
  line L40 (27.471, -55.971) -> (18.4788, -64.9632)
  line L41 (20.0067, -66.4933) -> (29, -57.5)
  line L42 (29, -57.5) -> (29, -75.5)
  line L43 (27.471, -55.971) -> (9.5, -55.971)
  line L44 (6.5, -55.971) -> (0.0001, -55.971)
  line L45 (29.1311, -53.1497) -> (18.1317, -53.2075)
  line L46 (15, -52.971) -> (0.0001, -52.971)
  line L47 (24.423, -16.955) -> (18, -16.955)
  line L48 (15, -16.9999) -> (0.0001, -16.9999)
  line L49 (22.0008, -106.476) -> (22.0008, -96.471)
  line L50 (19.0008, -106.476) -> (19.0008, -96.471)
  line L51 (3.5, -106.476) -> (3.5, -96.471)
  line L52 (6.5, -106.476) -> (6.5, -96.471)
  line L53 (6.5, -106.476) -> (19.0008, -106.476)
  line L54 (22.0008, -96.471) -> (29, -96.471)
  line L55 (19.0008, -96.471) -> (6.5, -96.471)
  line L56 (18, -28.1451) -> (18.1317, -53.2075)
  line L57 (15, -28) -> (15, -52.971)
  line L58 (43.2847, -28.1039) -> (29.9986, -51.0238)
  line L59 (-15.5021, -107.976) -> (-12.7423, -110.1593)
  line L60 (-12.7423, -110.1593) -> (-9.901, -107.976)
  line L61 (-33.999, -103.2094) -> (-33.999, -105.2276)
  line L62 (-33.999, -105.2276) -> (-30.7514, -108.4752)
  line L63 (-24.999, -101.4702) -> (-24.999, -106.4702)
  line L64 (-6.4997, -106.476) -> (-19.0005, -106.476)
  line L65 (-19.0005, -106.476) -> (-19.0005, -96.471)
  line L66 (-6.4997, -106.476) -> (-6.4997, -96.471)
  line L67 (-3.4997, -106.476) -> (-3.4997, -96.471)
  line L68 (-19.0005, -96.471) -> (-6.4997, -96.471)
  line L69 (-6.5069, -114.9941) -> (-11.0727, -111.4802)
  line L70 (-13.1987, -114.9663) -> (-15.5687, -114.9604)
  line L71 (-13.1987, -114.9663) -> (-9.9267, -114.9744)
  line L72 (-18.9776, -107.976) -> (-14.4459, -111.4803)
  line L73 (-14.4459, -111.4803) -> (-18.9776, -114.9744)
  line L74 (-18.9776, -107.976) -> (-18.9776, -114.9744)
  line L75 (-3.4997, -108.0056) -> (-3.4997, -115.0056)
  line L76 (-12.7464, -112.7943) -> (-15.5687, -114.9604)
  line L77 (-9.9267, -114.9744) -> (-13.4909, -114.9744) construction
  line L78 (-9.9267, -114.9744) -> (-12.7464, -112.7943)
  line L79 (-6.5069, -107.9759) -> (-6.5069, -114.9941)
  line L80 (-11.0727, -111.4802) -> (-6.5069, -107.9759)
  line L81 (-24.999, -101.4702) -> (-29.999, -101.4702)
  line L82 (-29.999, -101.4702) -> (-29.999, -106.4702)
  line L83 (-29.999, -106.4702) -> (-24.999, -106.4702)
  line L84 (-30.7514, -108.4752) -> (-29.2514, -109.9752)
  line L85 (-33.999, -103.2094) -> (-28.9997, -98.2258)
  line L86 (-25.4997, -109.9752) -> (-29.2514, -109.9752)
  line L87 (-22.0005, -114.4744) -> (-24.9996, -111.4752)
  line L88 (-22.0005, -108.476) -> (-22.0005, -114.4744)
  line L89 (-23.9996, -108.4752) -> (-25.4997, -109.9752)
  line L90 (-22.0005, -108.476) -> (-24.9996, -111.4752)
  line L91 (-22.0005, -106.476) -> (-23.9996, -108.4752)
  line L92 (-22.0005, -106.476) -> (-22.0005, -96.471)
  line L93 (-22.0005, -96.471) -> (-28.9997, -96.471)
  line L94 (-28.9997, -98.2258) -> (-28.9997, -96.471)
  circle A4 centre (-23.9996, -83) radius 1.5
  line L95 (-18.5053, -67.9945) -> (-27.4975, -77.0001)
  line L96 (-20.0064, -66.4933) -> (-28.9997, -75.5)
  line L97 (-28.9997, -57.5) -> (-28.9997, -75.5)
  line L98 (-20.0064, -66.4933) -> (-28.9997, -57.5)
  line L99 (-27.4707, -55.971) -> (-18.4785, -64.9632)
  line L100 (-27.4707, -55.971) -> (-9.4997, -55.971)
  line L101 (-9.4997, -55.971) -> (-18.4785, -64.9632)
  line L102 (-7.9986, -57.4721) -> (-16.9986, -66.4855)
  line L103 (-6.4997, -55.971) -> (0.0001, -55.971)
  line L104 (-51.4218, -5.197) -> (-51.4218, -13.955)
  line L105 (-48.1799, -1.9551) -> (-51.4218, -5.197)
  line L106 (-26.544, -16.0763) -> (-40.6652, -1.9551)
  line L107 (-40.6652, -1.9551) -> (-48.1799, -1.9551)
  line L108 (-24.4227, -16.955) -> (-26.544, -16.0763)
  circle A5 centre (-39.4723, -5.9876) radius 1.1
  circle A6 centre (-30.4214, -15.0386) radius 1.1
  line L109 (-24.4227, -16.955) -> (-17.9997, -16.955)
  line L110 (-51.4218, -13.955) -> (-45.0449, -25)
  line L111 (-29.8784, -50.8497) -> (-28.9997, -52.971)
  line L112 (0.0001, -13.9999) -> (-2.9999, -13.9999) construction
  circle A7 centre (-23.9996, -27) radius 1.5
  line L113 (-28.9997, -52.971) -> (-17.9997, -52.971)
  line L114 (-14.9997, -52.971) -> (0.0001, -52.971)
  line L115 (-14.9997, -28) -> (-14.9997, -52.971)
  line L116 (-17.9997, -28) -> (-17.9997, -52.971)
  line L117 (-43.2848, -28) -> (-29.8784, -50.8497)
  line L118 (-14.9997, -16.9999) -> (0.0001, -16.9999)
  line L119 (54.5012, -13.9979) -> (54.4973, -13.9973)
  line L120 (3.5, -115.0056) -> (-3.4997, -115.0056)
  line L121 (3.5, -96.471) -> (-3.4997, -96.471)
  line L122 (49.5, 1) -> (56.57, 1) construction
  line L123 (-49.4997, 1) -> (-56.5697, 1) construction
  line L124 (-15.5021, -107.976) -> (-9.901, -107.976)
  line L125 (15.5025, -107.9762) -> (9.9014, -107.9762)
  line L126 (-17.9997, -21) -> (-47.3543, -21)
  line L127 (-17.9997, -16.955) -> (-17.9997, -21)
  line L128 (-14.9997, -16.9999) -> (-14.9997, -21)
  line L129 (15, -21) -> (-14.9997, -21)
  line L130 (15, -16.9999) -> (15, -21)
  line L131 (18, -21) -> (18, -16.955)
  line L132 (18, -21) -> (47.3546, -21)
  line L133 (51.4221, -13.955) -> (47.3546, -21)
  line L134 (45.6012, -24.0917) -> (43.2847, -28.1039)
  line L135 (18, -28.1451) -> (18, -24.0917)
  line L136 (-17.9997, -24) -> (-45.6223, -24)
  line L137 (15, -24) -> (15, -28)
  line L138 (-14.9997, -24) -> (-14.9997, -28)
  line L139 (-17.9997, -28) -> (-17.9997, -24)
  circle A8 centre (-46.9997, -6.5) radius 2
  circle A9 centre (47, -6.5) radius 2
  circle A10 centre (-23.9996, -27) radius 3
  arc A11 (-21.0442, -83.5154) -> (-23.4842, -85.9554) centre (-23.9996, -83) ccw
  arc A12 (23.2638, -24.0917) -> (24.7361, -24.0917) centre (23.9999, -27) ccw
  arc A13 (23.4849, -85.9555) -> (21.0445, -83.515) centre (23.9999, -83) ccw
  circle A14 centre (30.4217, -15.0386) radius 2
  circle A15 centre (39.4726, -5.9876) radius 2
  circle A16 centre (-30.4214, -15.0386) radius 2
  circle A17 centre (-39.4723, -5.9876) radius 2
  line L140 (1, -29) -> (1, -42.9373)
  line L141 (-1, -29) -> (-1, -42.9372)
  line L142 (0, -50.9997) -> (-3.9281, -44.1961)
  line L143 (0, -50.9997) -> (3.9287, -44.1961)
  line L144 (-45.0449, -25) -> (-43.2848, -28)
  line L145 (-14.9997, -24) -> (15, -24)
  line L146 (-3.4997, -106.476) -> (3.5, -106.476)
  line L147 (-3.4997, -108.0056) -> (3.5, -108.0056)
  arc A18 (-9.367, -31.4996) -> (9.3679, -31.5004) centre (0.0001, -39) ccw
  arc A19 (-9.367, -31.4996) -> (-3.9281, -44.1961) centre (0.0003, -35) ccw
  arc A20 (3.9287, -44.1961) -> (9.3679, -31.5004) centre (0.0003, -35) ccw
  line L148 (-1, -29) -> (-1, -27.0628)
  line L149 (1, -29) -> (1, -27.0627)
  arc A21 (1, -42.9373) -> (1, -27.0627) centre (0.0003, -35) ccw
  arc A22 (-1, -27.0628) -> (-1, -42.9372) centre (0.0003, -35) ccw
  line L150 (49.5, 1) -> (39.5, 1)
  line L151 (49.5, 1) -> (54.5012, -3.9973)
  line L152 (54.5012, -3.9973) -> (54.5012, -13.9979)
  line L153 (-49.4997, 1) -> (-39.4997, 1)
  line L154 (-39.4997, 1) -> (-24.4999, -13.9998)
  line L155 (-24.4999, -13.9998) -> (0.0001, -13.9998)
  line L156 (-31.999, -96.471) -> (-36.9986, -101.4706)
  line L157 (-36.9986, -106.4763) -> (-31.9993, -111.4756)
  line L158 (-36.9986, -106.4763) -> (-36.9986, -101.4706)
  line L159 (-22.0002, -116.4747) -> (0.0003, -116.4747)
  line L160 (-31.9993, -111.4756) -> (-30.4993, -112.9756)
  line L161 (-30.4993, -112.9756) -> (-25.4993, -112.9756)
  line L162 (-25.4993, -112.9756) -> (-22.0002, -116.4747)
  line L163 (39.5, 1) -> (24.5001, -13.9998)
  line L164 (24.5001, -13.9998) -> (0.0001, -13.9998)
  line L165 (32.0002, -111.4756) -> (30.5003, -112.9756)
  line L166 (30.5003, -112.9756) -> (25.5003, -112.9756)
  line L167 (25.5003, -112.9756) -> (22.0011, -116.4747)
  line L168 (54.5012, -13.9979) -> (32.0031, -52.971)
  line L169 (32.0031, -96.471) -> (37.0024, -101.4702)
  line L170 (37.0024, -106.4734) -> (32.0002, -111.4756)
  line L171 (37.0024, -106.4734) -> (37.0024, -101.4702)
  line L172 (22.0011, -116.4747) -> (0.0003, -116.4747)
  line L173 (-49.4997, 1) -> (-54.499, -3.9992)
  line L174 (-54.499, -3.9992) -> (-54.499, -13.9998)
  line L175 (-54.499, -13.9998) -> (-31.999, -52.971)
  line L176 (-31.999, -52.971) -> (-31.999, -96.471)
  line L177 (32.0031, -52.971) -> (32.0031, -96.471)
  line L178 (29, -78.5022) -> (29, -91.4705)
  line L179 (-28.9997, -78.5045) -> (-28.9997, -91.4709)
  line L180 (-27.4975, -77.0001) -> (-28.9997, -78.5045)
  line L181 (-28.0288, -93.5) -> (28.0295, -93.5)
  line L182 (27.4978, -77) -> (29, -78.5022)
  line L183 (23.4849, -85.9555) -> (29, -91.4705)
  line L184 (-23.4842, -85.9554) -> (-28.9997, -91.4709)
  line L185 (-10.5143, -75.9855) -> (-28.0288, -93.5)
  line L186 (-16.9986, -66.4855) -> (-10.4934, -72.9645)
  line L187 (-8.9904, -74.4615) -> (-6.4417, -77)
  line L188 (-12.0144, -74.4855) -> (-21.0442, -83.5154)
  line L189 (-9.4997, -77.0001) -> (-10.5143, -75.9855)
  line L190 (-12.0144, -74.4855) -> (-18.5053, -67.9945)
  line L191 (-7.9986, -57.4721) -> (-1.4998, -63.9709)
  line L192 (6.5, -55.971) -> (0.0002, -62.4709)
  line L193 (-1.4998, -63.9709) -> (-10.4934, -72.9645)
  line L194 (-6.4997, -55.971) -> (0.0002, -62.4709)
  line L195 (7.9989, -57.4721) -> (1.5002, -63.9709)
  line L196 (0.0002, -65.4709) -> (-8.9904, -74.4615)
  line L197 (16.9989, -66.4855) -> (10.4938, -72.9644)
  line L198 (8.9908, -74.4614) -> (6.442, -77)
  line L199 (9.5, -77) -> (10.5147, -75.9853)
  line L200 (12.0147, -74.4853) -> (18.5056, -67.9944)
  line L201 (0.0002, -65.4709) -> (8.9908, -74.4614)
  line L202 (10.5147, -75.9853) -> (28.0295, -93.5)
  line L203 (1.5002, -63.9709) -> (10.4938, -72.9644)
  line L204 (12.0147, -74.4853) -> (21.0445, -83.515)
  line L205 (-6.4417, -77) -> (0.0002, -83.4419)
  line L206 (1.5292, -84.9709) -> (10.0584, -93.5)
  line L207 (-9.4997, -77.0001) -> (-1.5289, -84.9709)
  line L208 (0.0002, -86.4999) -> (7.0003, -93.5)
  line L209 (6.442, -77) -> (0.0002, -83.4419)
  line L210 (-1.5289, -84.9709) -> (-10.0579, -93.5)
  line L211 (9.5, -77) -> (1.5292, -84.9709)
  line L212 (0.0002, -86.4999) -> (-6.9999, -93.5)
  line L213 (18, -24.0917) -> (23.2638, -24.0917)
  line L214 (24.7361, -24.0917) -> (45.6012, -24.0917)
  point P0 (0, 0)
  constraints: 433 end point, 30 parallel, 23 centre point, 16 point on circle, 15 horizontal, 14 point on line, 13 perpendicular, 9 coincident, 8 vertical, 1 collinear, 1 equal length
extrude "Extrusion26" cut sketch "Sketch22" against normal blind 5 contours A0 | A1 | A5 | A6 | A8 | A9
sketch "Sketch23" plane through (0, 4, 0) normal (0, -1, 0) x (1, 0, 0)
  circle A0 centre (-47, -6.5) radius 3.5
  circle A1 centre (-47, -6.5) radius 2
  circle A2 centre (47, -6.5) radius 3.5
  circle A3 centre (47, -6.5) radius 2
  point P0 (0, 0)
  constraints: 4 centre point, 2 coincident
extrude "Extrusion27" add sketch "Sketch23" along normal blind 1
sketch "Sketch25" plane through (0, 0, 0) normal (0, -1, 0) x (1, 0, 0)
  line L0 (3.5, -115.0056) -> (3.5, -108.0056) projected
  line L1 (3.5, -108.0056) -> (-3.4997, -108.0056) projected
  line L2 (3.5, -115.0056) -> (-3.4997, -115.0056)
  line L3 (-3.4997, -115.0056) -> (-3.4997, -108.0056)
  line L4 (-3.4997, -108.0056) -> (3.5, -108.0056)
  line L5 (3.5, -108.0056) -> (3.5, -115.0056)
  line L6 (22.0011, -116.4748) -> (-22.0002, -116.4748) projected
  line L7 (-6.5, -96.471) -> (-6.5, -106.476) projected
  line L8 (6.5069, -116.4748) -> (-6.5, -116.4748)
  line L9 (-6.5, -116.4748) -> (-6.5, -106.476)
  line L10 (-6.5, -106.476) -> (6.5069, -106.476)
  line L11 (6.5069, -106.476) -> (6.5069, -116.4748)
  point P0 (0, 0)
  constraints: 16 end point, 4 parallel, 2 horizontal, 2 perpendicular, 1 point on line
extrude "Extrusion29" add sketch "Sketch25" along normal blind 10
sketch "Sketch26" plane through (-6.5, 0, -116.4748) normal (-1, 0, 0) x (0, 0, 1)
  line L0 (9.9987, 0) -> (9.9987, -10) projected
  line L1 (20.0038, 0) -> (9.9987, 0) projected
  line L2 (9.9987, -10) -> (20.0038, 0)
  line L3 (20.0038, 0) -> (9.9987, 0)
  line L4 (9.9987, 0) -> (9.9987, -10)
  point P0 (116.4748, 0)
  constraints: 6 end point, 2 perpendicular
extrude "Extrusion30" add sketch "Sketch26" against normal blind 3